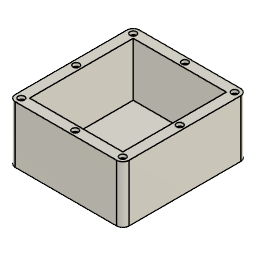
Case_Bottom (Autodesk Fusion 360 design; units mm, degrees)
part number: 2026-03-26-15-59-33-512
Autodesk Fusion 360 part; units mm, degrees
sketch "Sketch1" plane through (0, 0, 0) normal (0, 0, 1) x (1, 0, 0)
  line L0 (-39.1988, 50) -> (50.8012, 50)
  line L1 (50.8012, 50) -> (50.8012, -50)
  line L2 (50.8012, -50) -> (-39.1988, -50)
  line L3 (-39.1988, -50) -> (-39.1988, 50)
  line L4 (-43.1988, -60) -> (54.8012, -60)
  line L5 (60.8012, -54) -> (60.8012, 54)
  line L6 (54.8012, 60) -> (-43.1988, 60)
  line L7 (-49.1988, 54) -> (-49.1988, -54)
  circle A0 centre (9.8012, -55) radius 3.1
  circle A1 centre (54.8012, -54) radius 3.1
  circle A2 centre (-43.1988, -54) radius 3.1
  circle A3 centre (55.8012, 0) radius 3.1
  circle A4 centre (54.8012, 54) radius 3.1
  circle A5 centre (-44.1988, 0) radius 3.1
  circle A6 centre (-43.1988, 54) radius 3.1
  circle A7 centre (5.8012, 55) radius 3.1
  arc A8 (-49.1988, -54) -> (-43.1988, -60) centre (-43.1988, -54) ccw
  arc A9 (54.8012, -60) -> (60.8012, -54) centre (54.8012, -54) ccw
  arc A10 (60.8012, 54) -> (54.8012, 60) centre (54.8012, 54) ccw
  arc A11 (-43.1988, 60) -> (-49.1988, 54) centre (-43.1988, 54) ccw
  dimension "d1" = 90
  dimension "d5" = 10
  dimension "d6" = 10
  dimension "d7" = 6.2
  dimension "d8" = 6.2
  dimension "d9" = 6.2
  dimension "d10" = 6
  dimension "d11" = 6
  dimension "d12" = 6
  dimension "d13" = 6
  dimension "d14" = 59
  dimension "d15" = 6.2
  dimension "d16" = 6.2
  dimension "d17" = 6
  dimension "d18" = 6
  dimension "d19" = 60
  dimension "d20" = 6.2
  dimension "d21" = 5
  dimension "d22" = 5
  dimension "d23" = 5
  dimension "d24" = 6.2
  dimension "d25" = 6
  dimension "d26" = 6
  dimension "d27" = 60
  dimension "d28" = 6.2
  dimension "d29" = 5
  dimension "d30" = 55
  dimension "d31" = 6
  dimension "d32" = 6
  dimension "d33" = 6
  dimension "d34" = 6
  constraint horizontal L0
  constraint vertical L1
  constraint horizontal L2
  constraint vertical L3
  constraint tangent L4 A8
  constraint tangent L7 A8
  constraint tangent L4 A9
  constraint tangent L5 A9
  constraint tangent L5 A10
  constraint tangent L6 A10
  constraint tangent L7 A11
  constraint tangent L6 A11
  measures "d1" distance of L0.start L0.end
  measures "d5" distance of L3 L7
  measures "d6" distance of L0 L6
  measures "d7" diameter of A0
  measures "d8" diameter of A1
  measures "d9" diameter of A2
  measures "d10" distance of L7 A2.centre
  measures "d11" distance of L4 A2.centre
  measures "d12" distance of L5 A1.centre
  measures "d13" distance of L4 A1.centre
  measures "d14" distance of L7 A0.centre
  measures "d15" diameter of A3
  measures "d16" diameter of A4
  measures "d17" distance of L6 A4.centre
  measures "d18" distance of L5 A4.centre
  measures "d19" distance of L6 A3.centre
  measures "d20" diameter of A5
  measures "d21" distance of L7 A5.centre
  measures "d22" distance of L2 A0.centre
  measures "d23" distance of L5 A3.centre
  measures "d24" diameter of A6
  measures "d25" distance of L7 A6.centre
  measures "d26" distance of L6 A6.centre
  measures "d27" distance of L4 A5.centre
  measures "d28" diameter of A7
  measures "d29" distance of L6 A7.centre
  measures "d30" distance of L5 A7.centre
  measures "d31" radius of A8
  measures "d32" radius of A9
  measures "d33" radius of A10
  measures "d34" radius of A11
extrude "Extrude1" add sketch "Sketch1" along normal blind 55
extrude "Extrude2" add sketch "Sketch1" along normal blind 3.2 contours L0 L1 L2 L3
extrude "Extrude3" add sketch "Sketch1" along normal blind 51.85 contours A0 | A1 | A2 | A3 | A4 | A5 | A6 | A7
